Autodesk Fusion 360 part; units mm, degrees
(part 7 of 10)
sketch "Sketch35" plane through (0, 0, 9) normal (0, 0, 1) x (-1, 0, 0)
  line L0 (21, 35.9) -> (21, 34.9)
  line L1 (21, 34.9) -> (20, 34.9)
  line L2 (20, 34.9) -> (20, 35.9)
  line L3 (20, 35.9) -> (21, 35.9)
  line L4 (24, 35.9) -> (24, 34.9)
  line L5 (24, 34.9) -> (23, 34.9)
  line L6 (23, 34.9) -> (23, 35.9)
  line L7 (23, 35.9) -> (24, 35.9)
  line L8 (21, 33.27) -> (21, 32.27)
  line L9 (21, 32.27) -> (20, 32.27)
  line L10 (20, 32.27) -> (20, 33.27)
  line L11 (20, 33.27) -> (21, 33.27)
  line L12 (24, 33.27) -> (24, 32.27)
  line L13 (24, 32.27) -> (23, 32.27)
  line L14 (23, 32.27) -> (23, 33.27)
  line L15 (23, 33.27) -> (24, 33.27)
  line L16 (21, 30.64) -> (21, 29.64)
  line L17 (21, 29.64) -> (20, 29.64)
  line L18 (20, 29.64) -> (20, 30.64)
  line L19 (20, 30.64) -> (21, 30.64)
  line L20 (24, 30.64) -> (24, 29.64)
  line L21 (24, 29.64) -> (23, 29.64)
  line L22 (23, 29.64) -> (23, 30.64)
  line L23 (23, 30.64) -> (24, 30.64)
  line L24 (21, 28.01) -> (21, 27.01)
  line L25 (21, 27.01) -> (20, 27.01)
  line L26 (20, 27.01) -> (20, 28.01)
  line L27 (20, 28.01) -> (21, 28.01)
  line L28 (24, 28.01) -> (24, 27.01)
  line L29 (24, 27.01) -> (23, 27.01)
  line L30 (23, 27.01) -> (23, 28.01)
  line L31 (23, 28.01) -> (24, 28.01)
  line L32 (21, 25.38) -> (21, 24.38)
  line L33 (21, 24.38) -> (20, 24.38)
  line L34 (20, 24.38) -> (20, 25.38)
  line L35 (20, 25.38) -> (21, 25.38)
  line L36 (24, 25.38) -> (24, 24.38)
  line L37 (24, 24.38) -> (23, 24.38)
  line L38 (23, 24.38) -> (23, 25.38)
  line L39 (23, 25.38) -> (24, 25.38)
  line L40 (21, 18.05) -> (21, 17.05)
  line L41 (21, 17.05) -> (20, 17.05)
  line L42 (20, 17.05) -> (20, 18.05)
  line L43 (20, 18.05) -> (21, 18.05)
  line L44 (24, 15.42) -> (24, 14.42)
  line L45 (24, 14.42) -> (23, 14.42)
  line L46 (23, 14.42) -> (23, 15.42)
  line L47 (23, 15.42) -> (24, 15.42)
  line L48 (24, 18.05) -> (24, 17.05)
  line L49 (24, 17.05) -> (23, 17.05)
  line L50 (23, 17.05) -> (23, 18.05)
  line L51 (23, 18.05) -> (24, 18.05)
  line L52 (21, 15.42) -> (21, 14.42)
  line L53 (21, 14.42) -> (20, 14.42)
  line L54 (20, 14.42) -> (20, 15.42)
  line L55 (20, 15.42) -> (21, 15.42)
  line L56 (21, 20.68) -> (21, 19.68)
  line L57 (21, 19.68) -> (20, 19.68)
  line L58 (20, 19.68) -> (20, 20.68)
  line L59 (20, 20.68) -> (21, 20.68)
  line L60 (24, 12.79) -> (24, 11.79)
  line L61 (24, 11.79) -> (23, 11.79)
  line L62 (23, 11.79) -> (23, 12.79)
  line L63 (23, 12.79) -> (24, 12.79)
  line L64 (23, 20.68) -> (24, 20.68)
  line L65 (24, 20.68) -> (24, 19.68)
  line L66 (24, 19.68) -> (23, 19.68)
  line L67 (23, 19.68) -> (23, 20.68)
  line L68 (21, 12.79) -> (21, 11.79)
  line L69 (21, 11.79) -> (20, 11.79)
  line L70 (20, 11.79) -> (20, 12.79)
  line L71 (20, 12.79) -> (21, 12.79)
  line L72 (21, 9.16) -> (20, 9.16)
  line L73 (20, 9.16) -> (20, 10.16)
  line L74 (20, 10.16) -> (21, 10.16)
  line L75 (21, 10.16) -> (21, 9.16)
  line L76 (24, 10.16) -> (24, 9.16)
  line L77 (24, 9.16) -> (23, 9.16)
  line L78 (23, 9.16) -> (23, 10.16)
  line L79 (23, 10.16) -> (24, 10.16)
  line L80 (21, 5.46) -> (21, 4.46)
  line L81 (21, 4.46) -> (20, 4.46)
  line L82 (20, 4.46) -> (20, 5.46)
  line L83 (20, 5.46) -> (21, 5.46)
  line L84 (24, 5.46) -> (24, 4.46)
  line L85 (24, 4.46) -> (23, 4.46)
  line L86 (23, 4.46) -> (23, 5.46)
  line L87 (23, 5.46) -> (24, 5.46)
  line L88 (21, 2.83) -> (21, 1.83)
  line L89 (21, 1.83) -> (20, 1.83)
  line L90 (20, 1.83) -> (20, 2.83)
  line L91 (20, 2.83) -> (21, 2.83)
  line L92 (24, 2.83) -> (24, 1.83)
  line L93 (24, 1.83) -> (23, 1.83)
  line L94 (23, 1.83) -> (23, 2.83)
  line L95 (23, 2.83) -> (24, 2.83)
  line L96 (21, 0.2) -> (21, -0.8)
  line L97 (21, -0.8) -> (20, -0.8)
  line L98 (20, -0.8) -> (20, 0.2)
  line L99 (20, 0.2) -> (21, 0.2)
  line L100 (24, 0.2) -> (24, -0.8)
  line L101 (24, -0.8) -> (23, -0.8)
  line L102 (23, -0.8) -> (23, 0.2)
  line L103 (23, 0.2) -> (24, 0.2)
  line L104 (21, -2.43) -> (21, -3.43)
  line L105 (21, -3.43) -> (20, -3.43)
  line L106 (20, -3.43) -> (20, -2.43)
  line L107 (20, -2.43) -> (21, -2.43)
  line L108 (24, -2.43) -> (24, -3.43)
  line L109 (24, -3.43) -> (23, -3.43)
  line L110 (23, -3.43) -> (23, -2.43)
  line L111 (23, -2.43) -> (24, -2.43)
  line L112 (21, -5.06) -> (21, -6.06)
  line L113 (21, -6.06) -> (20, -6.06)
  line L114 (20, -6.06) -> (20, -5.06)
  line L115 (20, -5.06) -> (21, -5.06)
  line L116 (24, -5.06) -> (24, -6.06)
  line L117 (24, -6.06) -> (23, -6.06)
  line L118 (23, -6.06) -> (23, -5.06)
  line L119 (23, -5.06) -> (24, -5.06)
  line L120 (21, -9.76) -> (21, -10.76)
  line L121 (21, -10.76) -> (20, -10.76)
  line L122 (20, -10.76) -> (20, -9.76)
  line L123 (20, -9.76) -> (21, -9.76)
  line L124 (24, -9.76) -> (24, -10.76)
  line L125 (24, -10.76) -> (23, -10.76)
  line L126 (23, -10.76) -> (23, -9.76)
  line L127 (23, -9.76) -> (24, -9.76)
  line L128 (21, -12.39) -> (21, -13.39)
  line L129 (21, -13.39) -> (20, -13.39)
  line L130 (20, -13.39) -> (20, -12.39)
  line L131 (20, -12.39) -> (21, -12.39)
  line L132 (24, -12.39) -> (24, -13.39)
  line L133 (24, -13.39) -> (23, -13.39)
  line L134 (23, -13.39) -> (23, -12.39)
  line L135 (23, -12.39) -> (24, -12.39)
  line L136 (21, -15.02) -> (21, -16.02)
  line L137 (21, -16.02) -> (20, -16.02)
  line L138 (20, -16.02) -> (20, -15.02)
  line L139 (20, -15.02) -> (21, -15.02)
  line L140 (24, -15.02) -> (24, -16.02)
  line L141 (24, -16.02) -> (23, -16.02)
  line L142 (23, -16.02) -> (23, -15.02)
  line L143 (23, -15.02) -> (24, -15.02)
  line L144 (21, -17.65) -> (21, -18.65)
  line L145 (21, -18.65) -> (20, -18.65)
  line L146 (20, -18.65) -> (20, -17.65)
  line L147 (20, -17.65) -> (21, -17.65)
  line L148 (24, -17.65) -> (24, -18.65)
  line L149 (24, -18.65) -> (23, -18.65)
  line L150 (23, -18.65) -> (23, -17.65)
  line L151 (23, -17.65) -> (24, -17.65)
  line L152 (21, -20.28) -> (21, -21.28)
  line L153 (21, -21.28) -> (20, -21.28)
  line L154 (20, -21.28) -> (20, -20.28)
  line L155 (20, -20.28) -> (21, -20.28)
  line L156 (24, -20.28) -> (24, -21.28)
  line L157 (24, -21.28) -> (23, -21.28)
  line L158 (23, -21.28) -> (23, -20.28)
  line L159 (23, -20.28) -> (24, -20.28)
  line L160 (21, -24.98) -> (21, -25.98)
  line L161 (21, -25.98) -> (20, -25.98)
  line L162 (20, -25.98) -> (20, -24.98)
  line L163 (20, -24.98) -> (21, -24.98)
  line L164 (24, -24.98) -> (24, -25.98)
  line L165 (24, -25.98) -> (23, -25.98)
  line L166 (23, -25.98) -> (23, -24.98)
  line L167 (23, -24.98) -> (24, -24.98)
  line L168 (21, -27.61) -> (21, -28.61)
  line L169 (21, -28.61) -> (20, -28.61)
  line L170 (20, -28.61) -> (20, -27.61)
  line L171 (20, -27.61) -> (21, -27.61)
  line L172 (24, -27.61) -> (24, -28.61)
  line L173 (24, -28.61) -> (23, -28.61)
  line L174 (23, -28.61) -> (23, -27.61)
  line L175 (23, -27.61) -> (24, -27.61)
  line L176 (21, -30.24) -> (21, -31.24)
  line L177 (21, -31.24) -> (20, -31.24)
  line L178 (20, -31.24) -> (20, -30.24)
  line L179 (20, -30.24) -> (21, -30.24)
  line L180 (24, -30.24) -> (24, -31.24)
  line L181 (24, -31.24) -> (23, -31.24)
  line L182 (23, -31.24) -> (23, -30.24)
  line L183 (23, -30.24) -> (24, -30.24)
  line L184 (21, -32.87) -> (21, -33.87)
  line L185 (21, -33.87) -> (20, -33.87)
  line L186 (20, -33.87) -> (20, -32.87)
  line L187 (20, -32.87) -> (21, -32.87)
  line L188 (24, -32.87) -> (24, -33.87)
  line L189 (24, -33.87) -> (23, -33.87)
  line L190 (23, -33.87) -> (23, -32.87)
  line L191 (23, -32.87) -> (24, -32.87)
  line L192 (21, -35.5) -> (21, -36.5)
  line L193 (21, -36.5) -> (20, -36.5)
  line L194 (20, -36.5) -> (20, -35.5)
  line L195 (20, -35.5) -> (21, -35.5)
  line L196 (24, -35.5) -> (24, -36.5)
  line L197 (24, -36.5) -> (23, -36.5)
  line L198 (23, -36.5) -> (23, -35.5)
  line L199 (23, -35.5) -> (24, -35.5)
  line L200 (15.5, 38.77) -> (15.5, 37.77)
  line L201 (15.5, 37.77) -> (14.5, 37.77)
  line L202 (14.5, 37.77) -> (14.5, 38.77)
  line L203 (14.5, 38.77) -> (15.5, 38.77)
  line L204 (12.5, 38.77) -> (12.5, 37.77)
  line L205 (12.5, 37.77) -> (11.5, 37.77)
  line L206 (11.5, 37.77) -> (11.5, 38.77)
  line L207 (11.5, 38.77) -> (12.5, 38.77)
  line L208 (9.5, 38.77) -> (9.5, 37.77)
  line L209 (9.5, 37.77) -> (8.5, 37.77)
  line L210 (8.5, 37.77) -> (8.5, 38.77)
  line L211 (8.5, 38.77) -> (9.5, 38.77)
  line L212 (6.5, 38.77) -> (6.5, 37.77)
  line L213 (6.5, 37.77) -> (5.5, 37.77)
  line L214 (5.5, 37.77) -> (5.5, 38.77)
  line L215 (5.5, 38.77) -> (6.5, 38.77)
  line L216 (3.5, 38.77) -> (3.5, 37.77)
  line L217 (3.5, 37.77) -> (2.5, 37.77)
  line L218 (2.5, 37.77) -> (2.5, 38.77)
  line L219 (2.5, 38.77) -> (3.5, 38.77)
  line L220 (15.5, 36.14) -> (15.5, 35.14)
  line L221 (15.5, 35.14) -> (14.5, 35.14)
  line L222 (14.5, 35.14) -> (14.5, 36.14)
  line L223 (14.5, 36.14) -> (15.5, 36.14)
  line L224 (12.5, 36.14) -> (12.5, 35.14)
  line L225 (12.5, 35.14) -> (11.5, 35.14)
  line L226 (11.5, 35.14) -> (11.5, 36.14)
  line L227 (11.5, 36.14) -> (12.5, 36.14)
  line L228 (9.5, 36.14) -> (9.5, 35.14)
  line L229 (9.5, 35.14) -> (8.5, 35.14)
  line L230 (8.5, 35.14) -> (8.5, 36.14)
  line L231 (8.5, 36.14) -> (9.5, 36.14)
  line L232 (6.5, 36.14) -> (6.5, 35.14)
  line L233 (6.5, 35.14) -> (5.5, 35.14)
  line L234 (5.5, 35.14) -> (5.5, 36.14)
  line L235 (5.5, 36.14) -> (6.5, 36.14)
  line L236 (3.5, 36.14) -> (3.5, 35.14)
  line L237 (3.5, 35.14) -> (2.5, 35.14)
  line L238 (2.5, 35.14) -> (2.5, 36.14)
  line L239 (2.5, 36.14) -> (3.5, 36.14)
  line L240 (15.5, 33.51) -> (15.5, 32.51)
  line L241 (15.5, 32.51) -> (14.5, 32.51)
  line L242 (14.5, 32.51) -> (14.5, 33.51)
  line L243 (14.5, 33.51) -> (15.5, 33.51)
  line L244 (12.5, 33.51) -> (12.5, 32.51)
  line L245 (12.5, 32.51) -> (11.5, 32.51)
  line L246 (11.5, 32.51) -> (11.5, 33.51)
  line L247 (11.5, 33.51) -> (12.5, 33.51)
  line L248 (9.5, 33.51) -> (9.5, 32.51)
  line L249 (9.5, 32.51) -> (8.5, 32.51)
  line L250 (8.5, 32.51) -> (8.5, 33.51)
  line L251 (8.5, 33.51) -> (9.5, 33.51)
  line L252 (6.5, 33.51) -> (6.5, 32.51)
  line L253 (6.5, 32.51) -> (5.5, 32.51)
  line L254 (5.5, 32.51) -> (5.5, 33.51)
  line L255 (5.5, 33.51) -> (6.5, 33.51)
  line L256 (3.5, 33.51) -> (3.5, 32.51)
  line L257 (3.5, 32.51) -> (2.5, 32.51)
  line L258 (2.5, 32.51) -> (2.5, 33.51)
  line L259 (2.5, 33.51) -> (3.5, 33.51)
  line L260 (15.5, 30.88) -> (15.5, 29.88)
  line L261 (15.5, 29.88) -> (14.5, 29.88)
  line L262 (14.5, 29.88) -> (14.5, 30.88)
  line L263 (14.5, 30.88) -> (15.5, 30.88)
  line L264 (12.5, 30.88) -> (12.5, 29.88)
  line L265 (12.5, 29.88) -> (11.5, 29.88)
  line L266 (11.5, 29.88) -> (11.5, 30.88)
  line L267 (11.5, 30.88) -> (12.5, 30.88)
  line L268 (9.5, 30.88) -> (9.5, 29.88)
  line L269 (9.5, 29.88) -> (8.5, 29.88)
  line L270 (8.5, 29.88) -> (8.5, 30.88)
  line L271 (8.5, 30.88) -> (9.5, 30.88)
  line L272 (6.5, 30.88) -> (6.5, 29.88)
  line L273 (6.5, 29.88) -> (5.5, 29.88)
  line L274 (5.5, 29.88) -> (5.5, 30.88)
  line L275 (5.5, 30.88) -> (6.5, 30.88)
  line L276 (3.5, 30.88) -> (3.5, 29.88)
  line L277 (3.5, 29.88) -> (2.5, 29.88)
  line L278 (2.5, 29.88) -> (2.5, 30.88)
  line L279 (2.5, 30.88) -> (3.5, 30.88)
  line L280 (15.5, 28.25) -> (15.5, 27.25)
  line L281 (15.5, 27.25) -> (14.5, 27.25)
  line L282 (14.5, 27.25) -> (14.5, 28.25)
  line L283 (14.5, 28.25) -> (15.5, 28.25)
  line L284 (12.5, 28.25) -> (12.5, 27.25)
  line L285 (12.5, 27.25) -> (11.5, 27.25)
  line L286 (11.5, 27.25) -> (11.5, 28.25)
  line L287 (11.5, 28.25) -> (12.5, 28.25)
  line L288 (9.5, 28.25) -> (9.5, 27.25)
  line L289 (9.5, 27.25) -> (8.5, 27.25)
  line L290 (8.5, 27.25) -> (8.5, 28.25)
  line L291 (8.5, 28.25) -> (9.5, 28.25)
  line L292 (6.5, 28.25) -> (6.5, 27.25)
  line L293 (6.5, 27.25) -> (5.5, 27.25)
  line L294 (5.5, 27.25) -> (5.5, 28.25)
  line L295 (5.5, 28.25) -> (6.5, 28.25)
  line L296 (3.5, 28.25) -> (3.5, 27.25)
  line L297 (3.5, 27.25) -> (2.5, 27.25)
  line L298 (2.5, 27.25) -> (2.5, 28.25)
  line L299 (2.5, 28.25) -> (3.5, 28.25)
  line L300 (15.5, 25.62) -> (15.5, 24.62)
  line L301 (15.5, 24.62) -> (14.5, 24.62)
  line L302 (14.5, 24.62) -> (14.5, 25.62)
  line L303 (14.5, 25.62) -> (15.5, 25.62)
  line L304 (12.5, 25.62) -> (12.5, 24.62)
  line L305 (12.5, 24.62) -> (11.5, 24.62)
  line L306 (11.5, 24.62) -> (11.5, 25.62)
  line L307 (11.5, 25.62) -> (12.5, 25.62)
  line L308 (9.5, 25.62) -> (9.5, 24.62)
  line L309 (9.5, 24.62) -> (8.5, 24.62)
  line L310 (8.5, 24.62) -> (8.5, 25.62)
  line L311 (8.5, 25.62) -> (9.5, 25.62)
  line L312 (6.5, 25.62) -> (6.5, 24.62)
  line L313 (6.5, 24.62) -> (5.5, 24.62)
  line L314 (5.5, 24.62) -> (5.5, 25.62)
  line L315 (5.5, 25.62) -> (6.5, 25.62)
  line L316 (3.5, 25.62) -> (3.5, 24.62)
  line L317 (3.5, 24.62) -> (2.5, 24.62)
  line L318 (2.5, 24.62) -> (2.5, 25.62)
  line L319 (2.5, 25.62) -> (3.5, 25.62)
  line L320 (15.5, 22.99) -> (15.5, 21.99)
  line L321 (15.5, 21.99) -> (14.5, 21.99)
  line L322 (14.5, 21.99) -> (14.5, 22.99)
  line L323 (14.5, 22.99) -> (15.5, 22.99)
  line L324 (12.5, 22.99) -> (12.5, 21.99)
  line L325 (12.5, 21.99) -> (11.5, 21.99)
  line L326 (11.5, 21.99) -> (11.5, 22.99)
  line L327 (11.5, 22.99) -> (12.5, 22.99)
  line L328 (9.5, 22.99) -> (9.5, 21.99)
  line L329 (9.5, 21.99) -> (8.5, 21.99)
  line L330 (8.5, 21.99) -> (8.5, 22.99)
  line L331 (8.5, 22.99) -> (9.5, 22.99)
  line L332 (6.5, 22.99) -> (6.5, 21.99)
  line L333 (6.5, 21.99) -> (5.5, 21.99)
  line L334 (5.5, 21.99) -> (5.5, 22.99)
  line L335 (5.5, 22.99) -> (6.5, 22.99)
  line L336 (3.5, 22.99) -> (3.5, 21.99)
  line L337 (3.5, 21.99) -> (2.5, 21.99)
  line L338 (2.5, 21.99) -> (2.5, 22.99)
  line L339 (2.5, 22.99) -> (3.5, 22.99)
  line L340 (15.5, 20.36) -> (15.5, 19.36)
  line L341 (15.5, 19.36) -> (14.5, 19.36)
  line L342 (14.5, 19.36) -> (14.5, 20.36)
  line L343 (14.5, 20.36) -> (15.5, 20.36)
  line L344 (12.5, 20.36) -> (12.5, 19.36)
  line L345 (12.5, 19.36) -> (11.5, 19.36)
  line L346 (11.5, 19.36) -> (11.5, 20.36)
  line L347 (11.5, 20.36) -> (12.5, 20.36)
  line L348 (9.5, 20.36) -> (9.5, 19.36)
  line L349 (9.5, 19.36) -> (8.5, 19.36)
  line L350 (8.5, 19.36) -> (8.5, 20.36)
  line L351 (8.5, 20.36) -> (9.5, 20.36)
  line L352 (6.5, 20.36) -> (6.5, 19.36)
  line L353 (6.5, 19.36) -> (5.5, 19.36)
  line L354 (5.5, 19.36) -> (5.5, 20.36)
  line L355 (5.5, 20.36) -> (6.5, 20.36)
  line L356 (3.5, 20.36) -> (3.5, 19.36)
  line L357 (3.5, 19.36) -> (2.5, 19.36)
  line L358 (2.5, 19.36) -> (2.5, 20.36)
  line L359 (2.5, 20.36) -> (3.5, 20.36)
  line L360 (15.5, 17.73) -> (15.5, 16.73)
  line L361 (15.5, 16.73) -> (14.5, 16.73)
  line L362 (14.5, 16.73) -> (14.5, 17.73)
  line L363 (14.5, 17.73) -> (15.5, 17.73)
  line L364 (12.5, 17.73) -> (12.5, 16.73)
  line L365 (12.5, 16.73) -> (11.5, 16.73)
  line L366 (11.5, 16.73) -> (11.5, 17.73)
  line L367 (11.5, 17.73) -> (12.5, 17.73)
  line L368 (9.5, 17.73) -> (9.5, 16.73)
  line L369 (9.5, 16.73) -> (8.5, 16.73)
  line L370 (8.5, 16.73) -> (8.5, 17.73)
  line L371 (8.5, 17.73) -> (9.5, 17.73)
  line L372 (6.5, 17.73) -> (6.5, 16.73)
  line L373 (6.5, 16.73) -> (5.5, 16.73)
  line L374 (5.5, 16.73) -> (5.5, 17.73)
  line L375 (5.5, 17.73) -> (6.5, 17.73)
  line L376 (3.5, 17.73) -> (3.5, 16.73)
  line L377 (3.5, 16.73) -> (2.5, 16.73)
  line L378 (2.5, 16.73) -> (2.5, 17.73)
  line L379 (2.5, 17.73) -> (3.5, 17.73)
  line L380 (15.5, 15.1) -> (15.5, 14.1)
  line L381 (15.5, 14.1) -> (14.5, 14.1)
  line L382 (14.5, 14.1) -> (14.5, 15.1)
  line L383 (14.5, 15.1) -> (15.5, 15.1)
  line L384 (12.5, 15.1) -> (12.5, 14.1)
  line L385 (12.5, 14.1) -> (11.5, 14.1)
  line L386 (11.5, 14.1) -> (11.5, 15.1)
  line L387 (11.5, 15.1) -> (12.5, 15.1)
  line L388 (9.5, 15.1) -> (9.5, 14.1)
  line L389 (9.5, 14.1) -> (8.5, 14.1)
  line L390 (8.5, 14.1) -> (8.5, 15.1)
  line L391 (8.5, 15.1) -> (9.5, 15.1)
  line L392 (6.5, 15.1) -> (6.5, 14.1)
  line L393 (6.5, 14.1) -> (5.5, 14.1)
  line L394 (5.5, 14.1) -> (5.5, 15.1)
  line L395 (5.5, 15.1) -> (6.5, 15.1)
  line L396 (3.5, 15.1) -> (3.5, 14.1)
  line L397 (3.5, 14.1) -> (2.5, 14.1)
  line L398 (2.5, 14.1) -> (2.5, 15.1)
  line L399 (2.5, 15.1) -> (3.5, 15.1)
  line L400 (15.5, 12.47) -> (15.5, 11.47)
  line L401 (15.5, 11.47) -> (14.5, 11.47)
  line L402 (14.5, 11.47) -> (14.5, 12.47)
  line L403 (14.5, 12.47) -> (15.5, 12.47)
  line L404 (12.5, 12.47) -> (12.5, 11.47)
  line L405 (12.5, 11.47) -> (11.5, 11.47)
  line L406 (11.5, 11.47) -> (11.5, 12.47)
  line L407 (11.5, 12.47) -> (12.5, 12.47)
  line L408 (9.5, 12.47) -> (9.5, 11.47)
  line L409 (9.5, 11.47) -> (8.5, 11.47)
  line L410 (8.5, 11.47) -> (8.5, 12.47)
  line L411 (8.5, 12.47) -> (9.5, 12.47)
  line L412 (6.5, 12.47) -> (6.5, 11.47)
  line L413 (6.5, 11.47) -> (5.5, 11.47)
  line L414 (5.5, 11.47) -> (5.5, 12.47)
  line L415 (5.5, 12.47) -> (6.5, 12.47)
  line L416 (3.5, 12.47) -> (3.5, 11.47)
  line L417 (3.5, 11.47) -> (2.5, 11.47)
  line L418 (2.5, 11.47) -> (2.5, 12.47)
  line L419 (2.5, 12.47) -> (3.5, 12.47)
  line L420 (15.5, 9.84) -> (15.5, 8.84)
  line L421 (15.5, 8.84) -> (14.5, 8.84)
  line L422 (14.5, 8.84) -> (14.5, 9.84)
  line L423 (14.5, 9.84) -> (15.5, 9.84)
  line L424 (12.5, 9.84) -> (12.5, 8.84)
  line L425 (12.5, 8.84) -> (11.5, 8.84)
  line L426 (11.5, 8.84) -> (11.5, 9.84)
  line L427 (11.5, 9.84) -> (12.5, 9.84)
  line L428 (9.5, 9.84) -> (9.5, 8.84)
  line L429 (9.5, 8.84) -> (8.5, 8.84)
  line L430 (8.5, 8.84) -> (8.5, 9.84)
  line L431 (8.5, 9.84) -> (9.5, 9.84)
  line L432 (6.5, 9.84) -> (6.5, 8.84)
  line L433 (6.5, 8.84) -> (5.5, 8.84)
  line L434 (5.5, 8.84) -> (5.5, 9.84)
  line L435 (5.5, 9.84) -> (6.5, 9.84)
  line L436 (3.5, 9.84) -> (3.5, 8.84)
  line L437 (3.5, 8.84) -> (2.5, 8.84)
  line L438 (2.5, 8.84) -> (2.5, 9.84)
  line L439 (2.5, 9.84) -> (3.5, 9.84)
  line L440 (15.5, 7.21) -> (15.5, 6.21)
  line L441 (15.5, 6.21) -> (14.5, 6.21)
  line L442 (14.5, 6.21) -> (14.5, 7.21)
  line L443 (14.5, 7.21) -> (15.5, 7.21)
  line L444 (12.5, 7.21) -> (12.5, 6.21)
  line L445 (12.5, 6.21) -> (11.5, 6.21)
  line L446 (11.5, 6.21) -> (11.5, 7.21)
  line L447 (11.5, 7.21) -> (12.5, 7.21)
  line L448 (9.5, 7.21) -> (9.5, 6.21)
  line L449 (9.5, 6.21) -> (8.5, 6.21)
  line L450 (8.5, 6.21) -> (8.5, 7.21)
  line L451 (8.5, 7.21) -> (9.5, 7.21)
  line L452 (6.5, 7.21) -> (6.5, 6.21)
  line L453 (6.5, 6.21) -> (5.5, 6.21)
  line L454 (5.5, 6.21) -> (5.5, 7.21)
  line L455 (5.5, 7.21) -> (6.5, 7.21)
  line L456 (3.5, 7.21) -> (3.5, 6.21)
  line L457 (3.5, 6.21) -> (2.5, 6.21)
  line L458 (2.5, 6.21) -> (2.5, 7.21)
  line L459 (2.5, 7.21) -> (3.5, 7.21)
  line L460 (15.5, 4.58) -> (15.5, 3.58)
  line L461 (15.5, 3.58) -> (14.5, 3.58)
  line L462 (14.5, 3.58) -> (14.5, 4.58)
  line L463 (14.5, 4.58) -> (15.5, 4.58)
  line L464 (12.5, 4.58) -> (12.5, 3.58)
  line L465 (12.5, 3.58) -> (11.5, 3.58)
  line L466 (11.5, 3.58) -> (11.5, 4.58)
  line L467 (11.5, 4.58) -> (12.5, 4.58)
  line L468 (9.5, 4.58) -> (9.5, 3.58)
  line L469 (9.5, 3.58) -> (8.5, 3.58)
  line L470 (8.5, 3.58) -> (8.5, 4.58)
  line L471 (8.5, 4.58) -> (9.5, 4.58)
  line L472 (6.5, 4.58) -> (6.5, 3.58)
  line L473 (6.5, 3.58) -> (5.5, 3.58)
  line L474 (5.5, 3.58) -> (5.5, 4.58)
  line L475 (5.5, 4.58) -> (6.5, 4.58)
  line L476 (3.5, 4.58) -> (3.5, 3.58)
  line L477 (3.5, 3.58) -> (2.5, 3.58)
  line L478 (2.5, 3.58) -> (2.5, 4.58)
  line L479 (2.5, 4.58) -> (3.5, 4.58)
  line L480 (15.5, 1.95) -> (15.5, 0.95)
  line L481 (15.5, 0.95) -> (14.5, 0.95)
  line L482 (14.5, 0.95) -> (14.5, 1.95)
  line L483 (14.5, 1.95) -> (15.5, 1.95)
  line L484 (12.5, 1.95) -> (12.5, 0.95)
  line L485 (12.5, 0.95) -> (11.5, 0.95)
  line L486 (11.5, 0.95) -> (11.5, 1.95)
  line L487 (11.5, 1.95) -> (12.5, 1.95)
  line L488 (9.5, 1.95) -> (9.5, 0.95)
  line L489 (9.5, 0.95) -> (8.5, 0.95)
  line L490 (8.5, 0.95) -> (8.5, 1.95)
  line L491 (8.5, 1.95) -> (9.5, 1.95)
  line L492 (6.5, 1.95) -> (6.5, 0.95)
  line L493 (6.5, 0.95) -> (5.5, 0.95)
  line L494 (5.5, 0.95) -> (5.5, 1.95)
  line L495 (5.5, 1.95) -> (6.5, 1.95)
  line L496 (3.5, 1.95) -> (3.5, 0.95)
  line L497 (3.5, 0.95) -> (2.5, 0.95)
  line L498 (2.5, 0.95) -> (2.5, 1.95)
  line L499 (2.5, 1.95) -> (3.5, 1.95)
  line L500 (15.5, -0.68) -> (15.5, -1.68)
  line L501 (15.5, -1.68) -> (14.5, -1.68)
  line L502 (14.5, -1.68) -> (14.5, -0.68)
  line L503 (14.5, -0.68) -> (15.5, -0.68)
  line L504 (12.5, -0.68) -> (12.5, -1.68)
  line L505 (12.5, -1.68) -> (11.5, -1.68)
  line L506 (11.5, -1.68) -> (11.5, -0.68)
  line L507 (11.5, -0.68) -> (12.5, -0.68)
  line L508 (9.5, -0.68) -> (9.5, -1.68)
  line L509 (9.5, -1.68) -> (8.5, -1.68)
  line L510 (8.5, -1.68) -> (8.5, -0.68)
  line L511 (8.5, -0.68) -> (9.5, -0.68)
  line L512 (6.5, -0.68) -> (6.5, -1.68)
  line L513 (6.5, -1.68) -> (5.5, -1.68)
  line L514 (5.5, -1.68) -> (5.5, -0.68)
  line L515 (5.5, -0.68) -> (6.5, -0.68)
  line L516 (3.5, -0.68) -> (3.5, -1.68)
  line L517 (3.5, -1.68) -> (2.5, -1.68)
  line L518 (2.5, -1.68) -> (2.5, -0.68)
  line L519 (2.5, -0.68) -> (3.5, -0.68)
  line L520 (15.5, -3.31) -> (15.5, -4.31)
  line L521 (15.5, -4.31) -> (14.5, -4.31)
  line L522 (14.5, -4.31) -> (14.5, -3.31)
  line L523 (14.5, -3.31) -> (15.5, -3.31)
  line L524 (12.5, -3.31) -> (12.5, -4.31)
  line L525 (12.5, -4.31) -> (11.5, -4.31)
  line L526 (11.5, -4.31) -> (11.5, -3.31)
  line L527 (11.5, -3.31) -> (12.5, -3.31)
  line L528 (9.5, -3.31) -> (9.5, -4.31)
  line L529 (9.5, -4.31) -> (8.5, -4.31)
  line L530 (8.5, -4.31) -> (8.5, -3.31)
  line L531 (8.5, -3.31) -> (9.5, -3.31)
  line L532 (6.5, -3.31) -> (6.5, -4.31)
  line L533 (6.5, -4.31) -> (5.5, -4.31)
  line L534 (5.5, -4.31) -> (5.5, -3.31)
  line L535 (5.5, -3.31) -> (6.5, -3.31)
  line L536 (3.5, -3.31) -> (3.5, -4.31)
  line L537 (3.5, -4.31) -> (2.5, -4.31)
  line L538 (2.5, -4.31) -> (2.5, -3.31)
  line L539 (2.5, -3.31) -> (3.5, -3.31)
  line L540 (15.5, -5.94) -> (15.5, -6.94)
  line L541 (15.5, -6.94) -> (14.5, -6.94)
  line L542 (14.5, -6.94) -> (14.5, -5.94)
  line L543 (14.5, -5.94) -> (15.5, -5.94)
  line L544 (12.5, -5.94) -> (12.5, -6.94)
  line L545 (12.5, -6.94) -> (11.5, -6.94)
  line L546 (11.5, -6.94) -> (11.5, -5.94)
  line L547 (11.5, -5.94) -> (12.5, -5.94)
  line L548 (9.5, -5.94) -> (9.5, -6.94)
  line L549 (9.5, -6.94) -> (8.5, -6.94)
  line L550 (8.5, -6.94) -> (8.5, -5.94)
  line L551 (8.5, -5.94) -> (9.5, -5.94)
  line L552 (6.5, -5.94) -> (6.5, -6.94)
  line L553 (6.5, -6.94) -> (5.5, -6.94)
  line L554 (5.5, -6.94) -> (5.5, -5.94)
  line L555 (5.5, -5.94) -> (6.5, -5.94)
  line L556 (3.5, -5.94) -> (3.5, -6.94)
  line L557 (3.5, -6.94) -> (2.5, -6.94)
  line L558 (2.5, -6.94) -> (2.5, -5.94)
  line L559 (2.5, -5.94) -> (3.5, -5.94)
  line L560 (15.5, -8.57) -> (15.5, -9.57)
  line L561 (15.5, -9.57) -> (14.5, -9.57)
  line L562 (14.5, -9.57) -> (14.5, -8.57)
  line L563 (14.5, -8.57) -> (15.5, -8.57)
  line L564 (12.5, -8.57) -> (12.5, -9.57)
  line L565 (12.5, -9.57) -> (11.5, -9.57)
  line L566 (11.5, -9.57) -> (11.5, -8.57)
  line L567 (11.5, -8.57) -> (12.5, -8.57)
  line L568 (9.5, -8.57) -> (9.5, -9.57)
  line L569 (9.5, -9.57) -> (8.5, -9.57)
  line L570 (8.5, -9.57) -> (8.5, -8.57)
  line L571 (8.5, -8.57) -> (9.5, -8.57)
  line L572 (6.5, -8.57) -> (6.5, -9.57)
  line L573 (6.5, -9.57) -> (5.5, -9.57)
  line L574 (5.5, -9.57) -> (5.5, -8.57)
  line L575 (5.5, -8.57) -> (6.5, -8.57)
  line L576 (3.5, -8.57) -> (3.5, -9.57)
  line L577 (3.5, -9.57) -> (2.5, -9.57)
  line L578 (2.5, -9.57) -> (2.5, -8.57)
  line L579 (2.5, -8.57) -> (3.5, -8.57)
  line L580 (15.5, -11.2) -> (15.5, -12.2)
  line L581 (15.5, -12.2) -> (14.5, -12.2)
  line L582 (14.5, -12.2) -> (14.5, -11.2)
  line L583 (14.5, -11.2) -> (15.5, -11.2)
  line L584 (12.5, -11.2) -> (12.5, -12.2)
  line L585 (12.5, -12.2) -> (11.5, -12.2)
  line L586 (11.5, -12.2) -> (11.5, -11.2)
  line L587 (11.5, -11.2) -> (12.5, -11.2)
  line L588 (9.5, -11.2) -> (9.5, -12.2)
  line L589 (9.5, -12.2) -> (8.5, -12.2)
  line L590 (8.5, -12.2) -> (8.5, -11.2)
  line L591 (8.5, -11.2) -> (9.5, -11.2)
  line L592 (6.5, -11.2) -> (6.5, -12.2)
  line L593 (6.5, -12.2) -> (5.5, -12.2)
  line L594 (5.5, -12.2) -> (5.5, -11.2)
  line L595 (5.5, -11.2) -> (6.5, -11.2)
  line L596 (3.5, -11.2) -> (3.5, -12.2)
  line L597 (3.5, -12.2) -> (2.5, -12.2)
  line L598 (2.5, -12.2) -> (2.5, -11.2)
  line L599 (2.5, -11.2) -> (3.5, -11.2)
  line L600 (15.5, -13.83) -> (15.5, -14.83)
  line L601 (15.5, -14.83) -> (14.5, -14.83)
  line L602 (14.5, -14.83) -> (14.5, -13.83)
  line L603 (14.5, -13.83) -> (15.5, -13.83)
  line L604 (12.5, -13.83) -> (12.5, -14.83)
  line L605 (12.5, -14.83) -> (11.5, -14.83)
  line L606 (11.5, -14.83) -> (11.5, -13.83)
  line L607 (11.5, -13.83) -> (12.5, -13.83)
  line L608 (9.5, -13.83) -> (9.5, -14.83)
  line L609 (9.5, -14.83) -> (8.5, -14.83)
  line L610 (8.5, -14.83) -> (8.5, -13.83)
  line L611 (8.5, -13.83) -> (9.5, -13.83)
  line L612 (6.5, -13.83) -> (6.5, -14.83)
  line L613 (6.5, -14.83) -> (5.5, -14.83)
  line L614 (5.5, -14.83) -> (5.5, -13.83)
  line L615 (5.5, -13.83) -> (6.5, -13.83)
  line L616 (3.5, -13.83) -> (3.5, -14.83)
  line L617 (3.5, -14.83) -> (2.5, -14.83)
  line L618 (2.5, -14.83) -> (2.5, -13.83)
  line L619 (2.5, -13.83) -> (3.5, -13.83)
  line L620 (15.5, -16.46) -> (15.5, -17.46)
  line L621 (15.5, -17.46) -> (14.5, -17.46)
  line L622 (14.5, -17.46) -> (14.5, -16.46)
  line L623 (14.5, -16.46) -> (15.5, -16.46)
  line L624 (12.5, -16.46) -> (12.5, -17.46)
  line L625 (12.5, -17.46) -> (11.5, -17.46)
  line L626 (11.5, -17.46) -> (11.5, -16.46)
  line L627 (11.5, -16.46) -> (12.5, -16.46)
  line L628 (9.5, -16.46) -> (9.5, -17.46)
  line L629 (9.5, -17.46) -> (8.5, -17.46)
  line L630 (8.5, -17.46) -> (8.5, -16.46)
  line L631 (8.5, -16.46) -> (9.5, -16.46)
  line L632 (6.5, -16.46) -> (6.5, -17.46)
  line L633 (6.5, -17.46) -> (5.5, -17.46)
  line L634 (5.5, -17.46) -> (5.5, -16.46)
  line L635 (5.5, -16.46) -> (6.5, -16.46)
  line L636 (3.5, -16.46) -> (3.5, -17.46)
  line L637 (3.5, -17.46) -> (2.5, -17.46)
  line L638 (2.5, -17.46) -> (2.5, -16.46)
  line L639 (2.5, -16.46) -> (3.5, -16.46)
  line L640 (15.5, -19.09) -> (15.5, -20.09)
  line L641 (15.5, -20.09) -> (14.5, -20.09)
  line L642 (14.5, -20.09) -> (14.5, -19.09)
  line L643 (14.5, -19.09) -> (15.5, -19.09)
  line L644 (12.5, -19.09) -> (12.5, -20.09)
  line L645 (12.5, -20.09) -> (11.5, -20.09)
  line L646 (11.5, -20.09) -> (11.5, -19.09)
  line L647 (11.5, -19.09) -> (12.5, -19.09)
  line L648 (9.5, -19.09) -> (9.5, -20.09)
  line L649 (9.5, -20.09) -> (8.5, -20.09)
  line L650 (8.5, -20.09) -> (8.5, -19.09)
  line L651 (8.5, -19.09) -> (9.5, -19.09)
  line L652 (6.5, -19.09) -> (6.5, -20.09)
  line L653 (6.5, -20.09) -> (5.5, -20.09)
  line L654 (5.5, -20.09) -> (5.5, -19.09)
  line L655 (5.5, -19.09) -> (6.5, -19.09)
  line L656 (3.5, -19.09) -> (3.5, -20.09)
  line L657 (3.5, -20.09) -> (2.5, -20.09)
  line L658 (2.5, -20.09) -> (2.5, -19.09)
  line L659 (2.5, -19.09) -> (3.5, -19.09)
  line L660 (15.5, -21.72) -> (15.5, -22.72)
  line L661 (15.5, -22.72) -> (14.5, -22.72)
  line L662 (14.5, -22.72) -> (14.5, -21.72)
  line L663 (14.5, -21.72) -> (15.5, -21.72)
  line L664 (12.5, -21.72) -> (12.5, -22.72)
  line L665 (12.5, -22.72) -> (11.5, -22.72)
  line L666 (11.5, -22.72) -> (11.5, -21.72)
  line L667 (11.5, -21.72) -> (12.5, -21.72)
  line L668 (9.5, -21.72) -> (9.5, -22.72)
  line L669 (9.5, -22.72) -> (8.5, -22.72)
  line L670 (8.5, -22.72) -> (8.5, -21.72)
  line L671 (8.5, -21.72) -> (9.5, -21.72)
  line L672 (6.5, -21.72) -> (6.5, -22.72)
  line L673 (6.5, -22.72) -> (5.5, -22.72)
  line L674 (5.5, -22.72) -> (5.5, -21.72)
  line L675 (5.5, -21.72) -> (6.5, -21.72)
  line L676 (3.5, -21.72) -> (3.5, -22.72)
  line L677 (3.5, -22.72) -> (2.5, -22.72)
  line L678 (2.5, -22.72) -> (2.5, -21.72)
  line L679 (2.5, -21.72) -> (3.5, -21.72)
  line L680 (15.5, -24.35) -> (15.5, -25.35)
  line L681 (15.5, -25.35) -> (14.5, -25.35)
  line L682 (14.5, -25.35) -> (14.5, -24.35)
  line L683 (14.5, -24.35) -> (15.5, -24.35)
  line L684 (12.5, -24.35) -> (12.5, -25.35)
  line L685 (12.5, -25.35) -> (11.5, -25.35)
  line L686 (11.5, -25.35) -> (11.5, -24.35)
  line L687 (11.5, -24.35) -> (12.5, -24.35)
  line L688 (9.5, -24.35) -> (9.5, -25.35)
  line L689 (9.5, -25.35) -> (8.5, -25.35)
  line L690 (8.5, -25.35) -> (8.5, -24.35)
  line L691 (8.5, -24.35) -> (9.5, -24.35)
  line L692 (6.5, -24.35) -> (6.5, -25.35)
  line L693 (6.5, -25.35) -> (5.5, -25.35)
  line L694 (5.5, -25.35) -> (5.5, -24.35)
  line L695 (5.5, -24.35) -> (6.5, -24.35)
  line L696 (3.5, -24.35) -> (3.5, -25.35)
  line L697 (3.5, -25.35) -> (2.5, -25.35)
  line L698 (2.5, -25.35) -> (2.5, -24.35)
  line L699 (2.5, -24.35) -> (3.5, -24.35)
  line L700 (15.5, -26.98) -> (15.5, -27.98)
  line L701 (15.5, -27.98) -> (14.5, -27.98)
  line L702 (14.5, -27.98) -> (14.5, -26.98)
  line L703 (14.5, -26.98) -> (15.5, -26.98)
  line L704 (12.5, -26.98) -> (12.5, -27.98)
  line L705 (12.5, -27.98) -> (11.5, -27.98)
  line L706 (11.5, -27.98) -> (11.5, -26.98)
  line L707 (11.5, -26.98) -> (12.5, -26.98)
  line L708 (9.5, -26.98) -> (9.5, -27.98)
  line L709 (9.5, -27.98) -> (8.5, -27.98)
  line L710 (8.5, -27.98) -> (8.5, -26.98)
  line L711 (8.5, -26.98) -> (9.5, -26.98)
  line L712 (6.5, -26.98) -> (6.5, -27.98)
  line L713 (6.5, -27.98) -> (5.5, -27.98)
  line L714 (5.5, -27.98) -> (5.5, -26.98)
  line L715 (5.5, -26.98) -> (6.5, -26.98)
  line L716 (3.5, -26.98) -> (3.5, -27.98)
  line L717 (3.5, -27.98) -> (2.5, -27.98)
  line L718 (2.5, -27.98) -> (2.5, -26.98)
  line L719 (2.5, -26.98) -> (3.5, -26.98)
  line L720 (15.5, -29.61) -> (15.5, -30.61)
  line L721 (15.5, -30.61) -> (14.5, -30.61)
  line L722 (14.5, -30.61) -> (14.5, -29.61)
  line L723 (14.5, -29.61) -> (15.5, -29.61)
  line L724 (12.5, -29.61) -> (12.5, -30.61)
  line L725 (12.5, -30.61) -> (11.5, -30.61)
  line L726 (11.5, -30.61) -> (11.5, -29.61)
  line L727 (11.5, -29.61) -> (12.5, -29.61)
  line L728 (9.5, -29.61) -> (9.5, -30.61)
  line L729 (9.5, -30.61) -> (8.5, -30.61)
  line L730 (8.5, -30.61) -> (8.5, -29.61)
  line L731 (8.5, -29.61) -> (9.5, -29.61)
  line L732 (6.5, -29.61) -> (6.5, -30.61)
  line L733 (6.5, -30.61) -> (5.5, -30.61)
  line L734 (5.5, -30.61) -> (5.5, -29.61)
  line L735 (5.5, -29.61) -> (6.5, -29.61)
  line L736 (3.5, -29.61) -> (3.5, -30.61)
  line L737 (3.5, -30.61) -> (2.5, -30.61)
  line L738 (2.5, -30.61) -> (2.5, -29.61)
  line L739 (2.5, -29.61) -> (3.5, -29.61)
  line L740 (15.5, -32.24) -> (15.5, -33.24)
  line L741 (15.5, -33.24) -> (14.5, -33.24)
  line L742 (14.5, -33.24) -> (14.5, -32.24)
  line L743 (14.5, -32.24) -> (15.5, -32.24)
  line L744 (12.5, -32.24) -> (12.5, -33.24)
  line L745 (12.5, -33.24) -> (11.5, -33.24)
  line L746 (11.5, -33.24) -> (11.5, -32.24)
  line L747 (11.5, -32.24) -> (12.5, -32.24)
  line L748 (9.5, -32.24) -> (9.5, -33.24)
  line L749 (9.5, -33.24) -> (8.5, -33.24)
  line L750 (8.5, -33.24) -> (8.5, -32.24)
  line L751 (8.5, -32.24) -> (9.5, -32.24)
  line L752 (6.5, -32.24) -> (6.5, -33.24)
  line L753 (6.5, -33.24) -> (5.5, -33.24)
  line L754 (5.5, -33.24) -> (5.5, -32.24)
  line L755 (5.5, -32.24) -> (6.5, -32.24)
  line L756 (3.5, -32.24) -> (3.5, -33.24)
  line L757 (3.5, -33.24) -> (2.5, -33.24)
  line L758 (2.5, -33.24) -> (2.5, -32.24)
  line L759 (2.5, -32.24) -> (3.5, -32.24)
  line L760 (15.5, -34.87) -> (15.5, -35.87)
  line L761 (15.5, -35.87) -> (14.5, -35.87)
  line L762 (14.5, -35.87) -> (14.5, -34.87)
  line L763 (14.5, -34.87) -> (15.5, -34.87)
  line L764 (12.5, -34.87) -> (12.5, -35.87)
  line L765 (12.5, -35.87) -> (11.5, -35.87)
  line L766 (11.5, -35.87) -> (11.5, -34.87)
  line L767 (11.5, -34.87) -> (12.5, -34.87)
  line L768 (9.5, -34.87) -> (9.5, -35.87)
  line L769 (9.5, -35.87) -> (8.5, -35.87)
  line L770 (8.5, -35.87) -> (8.5, -34.87)
  line L771 (8.5, -34.87) -> (9.5, -34.87)
  line L772 (6.5, -34.87) -> (6.5, -35.87)
  line L773 (6.5, -35.87) -> (5.5, -35.87)
  line L774 (5.5, -35.87) -> (5.5, -34.87)
  line L775 (5.5, -34.87) -> (6.5, -34.87)
  line L776 (3.5, -34.87) -> (3.5, -35.87)
  line L777 (3.5, -35.87) -> (2.5, -35.87)
  line L778 (2.5, -35.87) -> (2.5, -34.87)
  line L779 (2.5, -34.87) -> (3.5, -34.87)
  line L780 (15.5, -37.5) -> (15.5, -38.5)
  line L781 (15.5, -38.5) -> (14.5, -38.5)
  line L782 (14.5, -38.5) -> (14.5, -37.5)
  line L783 (14.5, -37.5) -> (15.5, -37.5)
  line L784 (12.5, -37.5) -> (12.5, -38.5)
  line L785 (12.5, -38.5) -> (11.5, -38.5)
  line L786 (11.5, -38.5) -> (11.5, -37.5)
  line L787 (11.5, -37.5) -> (12.5, -37.5)
  line L788 (9.5, -37.5) -> (9.5, -38.5)
  line L789 (9.5, -38.5) -> (8.5, -38.5)
  line L790 (8.5, -38.5) -> (8.5, -37.5)
  line L791 (8.5, -37.5) -> (9.5, -37.5)
  line L792 (6.5, -37.5) -> (6.5, -38.5)
  line L793 (6.5, -38.5) -> (5.5, -38.5)
  line L794 (5.5, -38.5) -> (5.5, -37.5)
  line L795 (5.5, -37.5) -> (6.5, -37.5)
  line L796 (3.5, -37.5) -> (3.5, -38.5)
  line L797 (3.5, -38.5) -> (2.5, -38.5)
  line L798 (2.5, -38.5) -> (2.5, -37.5)
  line L799 (2.5, -37.5) -> (3.5, -37.5)
  line L800 (1, 40.5) -> (1, -40.5)
  line L801 (1, -40.5) -> (26.5, -40.5)
  line L802 (26.5, -40.5) -> (26.5, 40.5)
  line L803 (26.5, 40.5) -> (1, 40.5)
  line L804 (25, -36.5) -> (25.5, -36.5)
  line L805 (25.5, -36.5) -> (25.5, 36)
  line L806 (25.5, 36) -> (25, 36)
  line L807 (25, 36) -> (25, -36.5)
  line L808 (25, -36.5) -> (25.5, 36) construction
  line L809 (25.5, -36.5) -> (25, 36) construction
  point P0 (25.25, -0.25)
  dimension "d217" = 72.5
  dimension "d218" = 0.5
  dimension "d219" = 1
  constraint horizontal L804
  constraint perpendicular L804 L805
  constraint parallel L804 L806
  constraint parallel L805 L807
  constraint coincident L808 P0
  constraint coincident L809 P0
  measures "d217" distance of L804.end L805.end
  measures "d218" distance of L804.start L804.end
  measures "d219" distance of L802 L805
extrude "Extrude1'" add sketch "Sketch35" along normal blind 0.01 separate body contours L804 L805 L806 L807 makes body 2 in component "Component"